Autodesk Fusion 360 part; units mm, degrees
(part 3 of 3)
ref_plane "Piano di lavoro7" through (0, 0, 107.5) normal (0, 0, 1) x (1, 0, 0) in component "14_Guscio_mobile_cannone_removibile"
sketch "Schizzo12 (5)" plane through (0, 0, 107.5) normal (0, 0, 1) x (1, 0, 0) in component "14_Guscio_mobile_cannone_removibile"
  line L0 (-15, -13) -> (15, -13)
  line L1 (15, -13) -> (15, 2)
  line L2 (15, 2) -> (-15, 2)
  line L3 (-15, 2) -> (-15, -13)
extrude "Tasca_coperchio_culatta_a_filo" cut sketch "Schizzo12 (5)" along normal blind 2 bodies 30 in component "14_Guscio_mobile_cannone_removibile"
ref_plane "Piano di lavoro8" through (0, -6, 0) normal (0, 1, 0) x (0, 0, 1) in component "14_Guscio_mobile_cannone_removibile"
sketch "Schizzo13 (5)" plane through (0, -6, 0) normal (0, 1, 0) x (1, 0, 0) in component "14_Guscio_mobile_cannone_removibile"
  circle A0 centre (0, -96.5) radius 5.5
extrude "Estrusione_Guida_interna_culatta_manuale" add sketch "Schizzo13 (5)" along normal blind 8 separate body makes body 33 in component "14_Guscio_mobile_cannone_removibile"
ref_plane "Piano di lavoro9" through (0, -6, 0) normal (0, 1, 0) x (0, 0, 1) in component "14_Guscio_mobile_cannone_removibile"
sketch "Schizzo14 (5)" plane through (0, -6, 0) normal (0, 1, 0) x (1, 0, 0) in component "14_Guscio_mobile_cannone_removibile"
  circle A0 centre (0, -96.5) radius 4
extrude "Foro_coassiale_guida_culatta_manuale" cut sketch "Schizzo14 (5)" along normal blind 8 bodies 33 in component "14_Guscio_mobile_cannone_removibile"
ref_plane "Piano di lavoro10" through (0, 0, 100.8) normal (0, 0, 1) x (1, 0, 0) in component "14_Guscio_mobile_cannone_removibile"
sketch "Schizzo15 (5)" plane through (0, 0, 100.8) normal (0, 0, 1) x (1, 0, 0) in component "14_Guscio_mobile_cannone_removibile"
  line L0 (-2, -6) -> (2, -6)
  line L1 (2, -6) -> (2, 2)
  line L2 (2, 2) -> (-2, 2)
  line L3 (-2, 2) -> (-2, -6)
extrude "Estrusione_Nervatura_tetto_guida_culatta" add sketch "Schizzo15 (5)" along normal blind 6.4 bodies 30 33 in component "14_Guscio_mobile_cannone_removibile"
ref_plane "Piano di lavoro11" through (0, 0, 103) normal (0, 0, 1) x (1, 0, 0) in component "14_Guscio_mobile_cannone_removibile"
sketch "Schizzo16 (4)" plane through (0, 0, 103) normal (0, 0, 1) x (1, 0, 0) in component "14_Guscio_mobile_cannone_removibile"
  circle A0 centre (-10.75, -4) radius 3
extrude "Estrusione_Boss_M2_5_coperchio_culatta_01" add sketch "Schizzo16 (4)" along normal blind 4.2 bodies 30 in component "14_Guscio_mobile_cannone_removibile"
sketch "Schizzo17 (3)" plane through (0, 0, 103) normal (0, 0, 1) x (1, 0, 0) in component "14_Guscio_mobile_cannone_removibile"
  circle A0 centre (-10.75, -4) radius 1.1
extrude "Preforo_M2_5_coperchio_culatta_01" cut sketch "Schizzo17 (3)" along normal blind 4.6 bodies 30 in component "14_Guscio_mobile_cannone_removibile"
sketch "Schizzo18 (3)" plane through (0, 0, 103) normal (0, 0, 1) x (1, 0, 0) in component "14_Guscio_mobile_cannone_removibile"
  circle A0 centre (10.75, -4) radius 3
extrude "Estrusione_Boss_M2_5_coperchio_culatta_02" add sketch "Schizzo18 (3)" along normal blind 4.2 bodies 30 in component "14_Guscio_mobile_cannone_removibile"
sketch "Schizzo19 (3)" plane through (0, 0, 103) normal (0, 0, 1) x (1, 0, 0) in component "14_Guscio_mobile_cannone_removibile"
  circle A0 centre (10.75, -4) radius 1.1
extrude "Preforo_M2_5_coperchio_culatta_02" cut sketch "Schizzo19 (3)" along normal blind 4.6 bodies 30 in component "14_Guscio_mobile_cannone_removibile"
sketch "Schizzo20 (3)" plane through (0, 0, 83.5) normal (0, 0, 1) x (1, 0, 0) in component "14_Guscio_mobile_cannone_removibile"
  line L0 (-28, 40.5) -> (-5.5, 40.5)
  line L1 (-5.5, 40.5) -> (-5.5, 43)
  line L2 (-5.5, 43) -> (-28, 43)
  line L3 (-28, 43) -> (-28, 40.5)
extrude "Estrusione_Parete_mobile_Anteriore_Ovest" add sketch "Schizzo20 (3)" along normal blind 26 bodies 30 in component "14_Guscio_mobile_cannone_removibile"
sketch "Schizzo21 (3)" plane through (0, 0, 83.5) normal (0, 0, 1) x (1, 0, 0) in component "14_Guscio_mobile_cannone_removibile"
  line L0 (5.5, 40.5) -> (28, 40.5)
  line L1 (28, 40.5) -> (28, 43)
  line L2 (28, 43) -> (5.5, 43)
  line L3 (5.5, 43) -> (5.5, 40.5)
extrude "Estrusione_Parete_mobile_Anteriore_Est" add sketch "Schizzo21 (3)" along normal blind 26 bodies 30 in component "14_Guscio_mobile_cannone_removibile"
ref_plane "Piano di lavoro12" through (0, 0, 102) normal (0, 0, 1) x (1, 0, 0) in component "14_Guscio_mobile_cannone_removibile"
sketch "Schizzo22 (3)" plane through (0, 0, 102) normal (0, 0, 1) x (1, 0, 0) in component "14_Guscio_mobile_cannone_removibile"
  line L0 (-5.5, 40.5) -> (5.5, 40.5)
  line L1 (5.5, 40.5) -> (5.5, 43)
  line L2 (5.5, 43) -> (-5.5, 43)
  line L3 (-5.5, 43) -> (-5.5, 40.5)
extrude "Estrusione_Ponte_superiore_cava_U_canna" add sketch "Schizzo22 (3)" along normal blind 7.5 bodies 30 in component "14_Guscio_mobile_cannone_removibile"
ref_plane "Piano di lavoro13" through (0, -13, 0) normal (0, 1, 0) x (0, 0, 1) in component "14_Guscio_mobile_cannone_removibile"
sketch "Schizzo23 (3)" plane through (0, -13, 0) normal (0, 1, 0) x (1, 0, 0) in component "14_Guscio_mobile_cannone_removibile"
  line L0 (-3, -83.5) -> (3, -83.5)
  line L1 (3, -83.5) -> (3, -87.5)
  line L2 (3, -87.5) -> (-3, -87.5)
  line L3 (-3, -87.5) -> (-3, -83.5)
extrude "Tacca_posteriore_cavo_cannone_aperta_inferiormente" cut sketch "Schizzo23 (3)" along normal blind 2.5 bodies 30 in component "14_Guscio_mobile_cannone_removibile"
ref_plane "Piano di lavoro14" through (0, 0, 85.5) normal (0, 0, 1) x (1, 0, 0) in component "14_Guscio_mobile_cannone_removibile"
sketch "Schizzo24 (3)" plane through (0, 0, 85.5) normal (0, 0, 1) x (1, 0, 0) in component "14_Guscio_mobile_cannone_removibile"
  circle A0 centre (-20, -5) radius 5
extrude "Estrusione_Colonna_M3_guscio_mobile_01" add sketch "Schizzo24 (3)" along normal blind 21.7 bodies 30 in component "14_Guscio_mobile_cannone_removibile"
sketch "Schizzo25 (3)" plane through (0, 0, 85.5) normal (0, 0, 1) x (1, 0, 0) in component "14_Guscio_mobile_cannone_removibile"
  circle A0 centre (-20, -5) radius 1.75
extrude "Foro_M3_guscio_mobile_01" cut sketch "Schizzo25 (3)" along normal blind 24 bodies 30 in component "14_Guscio_mobile_cannone_removibile"
sketch "Schizzo26 (3)" plane through (0, 0, 85.5) normal (0, 0, 1) x (1, 0, 0) in component "14_Guscio_mobile_cannone_removibile"
  circle A0 centre (20, -5) radius 5
extrude "Estrusione_Colonna_M3_guscio_mobile_02" add sketch "Schizzo26 (3)" along normal blind 21.7 bodies 30 in component "14_Guscio_mobile_cannone_removibile"
sketch "Schizzo27 (3)" plane through (0, 0, 85.5) normal (0, 0, 1) x (1, 0, 0) in component "14_Guscio_mobile_cannone_removibile"
  circle A0 centre (20, -5) radius 1.75
extrude "Foro_M3_guscio_mobile_02" cut sketch "Schizzo27 (3)" along normal blind 24 bodies 30 in component "14_Guscio_mobile_cannone_removibile"
sketch "Schizzo28 (3)" plane through (0, 0, 85.5) normal (0, 0, 1) x (1, 0, 0) in component "14_Guscio_mobile_cannone_removibile"
  circle A0 centre (-20, 35) radius 5
extrude "Estrusione_Colonna_M3_guscio_mobile_03" add sketch "Schizzo28 (3)" along normal blind 21.7 bodies 30 in component "14_Guscio_mobile_cannone_removibile"
sketch "Schizzo29 (3)" plane through (0, 0, 85.5) normal (0, 0, 1) x (1, 0, 0) in component "14_Guscio_mobile_cannone_removibile"
  circle A0 centre (-20, 35) radius 1.75
extrude "Foro_M3_guscio_mobile_03" cut sketch "Schizzo29 (3)" along normal blind 24 bodies 30 in component "14_Guscio_mobile_cannone_removibile"
sketch "Schizzo30 (3)" plane through (0, 0, 85.5) normal (0, 0, 1) x (1, 0, 0) in component "14_Guscio_mobile_cannone_removibile"
  circle A0 centre (20, 35) radius 5
extrude "Estrusione_Colonna_M3_guscio_mobile_04" add sketch "Schizzo30 (3)" along normal blind 21.7 bodies 30 in component "14_Guscio_mobile_cannone_removibile"
sketch "Schizzo31 (3)" plane through (0, 0, 85.5) normal (0, 0, 1) x (1, 0, 0) in component "14_Guscio_mobile_cannone_removibile"
  circle A0 centre (20, 35) radius 1.75
extrude "Foro_M3_guscio_mobile_04" cut sketch "Schizzo31 (3)" along normal blind 24 bodies 30 in component "14_Guscio_mobile_cannone_removibile"
ref_plane "Piano di lavoro1" through (0, 0, 107.5) normal (0, 0, 1) x (1, 0, 0) in component "15_Coperchio_culatta_L_removibile_M2_5"
sketch "Schizzo1 (23)" plane through (0, 0, 107.5) normal (0, 0, 1) x (1, 0, 0) in component "15_Coperchio_culatta_L_removibile_M2_5"
  line L0 (-14.7, -12.7) -> (14.7, -12.7)
  line L1 (14.7, -12.7) -> (14.7, 1.7)
  line L2 (14.7, 1.7) -> (-14.7, 1.7)
  line L3 (-14.7, 1.7) -> (-14.7, -12.7)
extrude "Estrusione_Piastra_superiore_coperchio_culatta_a_filo" add sketch "Schizzo1 (23)" along normal blind 1.8 separate body makes body 34 in component "15_Coperchio_culatta_L_removibile_M2_5"
ref_plane "Piano di lavoro2" through (0, -12.7, 0) normal (0, 1, 0) x (0, 0, 1) in component "15_Coperchio_culatta_L_removibile_M2_5"
sketch "Schizzo2 (22)" plane through (0, -12.7, 0) normal (0, 1, 0) x (1, 0, 0) in component "15_Coperchio_culatta_L_removibile_M2_5"
  line L0 (-6.7, -90.8) -> (6.7, -90.8)
  line L1 (6.7, -90.8) -> (6.7, -109.2)
  line L2 (6.7, -109.2) -> (-6.7, -109.2)
  line L3 (-6.7, -109.2) -> (-6.7, -90.8)
extrude "Estrusione_Piastra_posteriore_coperchio_culatta" add sketch "Schizzo2 (22)" along normal blind 1.9 bodies 34 in component "15_Coperchio_culatta_L_removibile_M2_5"
ref_plane "Piano di lavoro3" through (0, 0, 108.1) normal (0, 0, 1) x (1, 0, 0) in component "15_Coperchio_culatta_L_removibile_M2_5"
ref_plane "Piano di lavoro4" through (0, 0, 109.3) normal (0, 0, 1) x (1, 0, 0) in component "15_Coperchio_culatta_L_removibile_M2_5"
sketch "Schizzo3 (21)" plane through (0, 0, 107.5) normal (0, 0, 1) x (1, 0, 0) in component "15_Coperchio_culatta_L_removibile_M2_5"
  circle A0 centre (-10.75, -4) radius 1.35
extrude "Foro_M2_5_coperchio_culatta_01" cut sketch "Schizzo3 (21)" along normal blind 1.8 bodies 34 in component "15_Coperchio_culatta_L_removibile_M2_5"
sketch "Schizzo4 (20)" plane through (0, 0, 108.1) normal (0, 0, 1) x (1, 0, 0) in component "15_Coperchio_culatta_L_removibile_M2_5"
  circle A0 centre (-10.75, -4) radius 1.35
sketch "Schizzo5 (12)" plane through (0, 0, 109.3) normal (0, 0, 1) x (1, 0, 0) in component "15_Coperchio_culatta_L_removibile_M2_5"
  circle A0 centre (-10.75, -4) radius 2.5
loft "Svasatura_M2_5_coperchio_culatta_01" cut profiles "Schizzo4 (20)", "Schizzo5 (12)" section 1 section 2 bodies 34 in component "15_Coperchio_culatta_L_removibile_M2_5"
sketch "Schizzo6 (10)" plane through (0, 0, 107.5) normal (0, 0, 1) x (1, 0, 0) in component "15_Coperchio_culatta_L_removibile_M2_5"
  circle A0 centre (10.75, -4) radius 1.35
extrude "Foro_M2_5_coperchio_culatta_02" cut sketch "Schizzo6 (10)" along normal blind 1.8 bodies 34 in component "15_Coperchio_culatta_L_removibile_M2_5"
sketch "Schizzo7 (8)" plane through (0, 0, 108.1) normal (0, 0, 1) x (1, 0, 0) in component "15_Coperchio_culatta_L_removibile_M2_5"
  circle A0 centre (10.75, -4) radius 1.35
sketch "Schizzo8 (8)" plane through (0, 0, 109.3) normal (0, 0, 1) x (1, 0, 0) in component "15_Coperchio_culatta_L_removibile_M2_5"
  circle A0 centre (10.75, -4) radius 2.5
loft "Svasatura_M2_5_coperchio_culatta_02" cut profiles "Schizzo7 (8)", "Schizzo8 (8)" section 1 section 2 bodies 34 in component "15_Coperchio_culatta_L_removibile_M2_5"
sketch "Schizzo1 (24)" plane through (0, 0, 0) normal (0, 1, 0) x (1, 0, 0)
  line L0 (0, -20) -> (0, 20)
ref_plane "Piano di lavoro1" through (0, 0, 81.5) normal (0, 0, 1) x (1, 0, 0)
sketch "Schizzo2 (23)" plane through (0, 0, 81.5) normal (0, 0, 1) x (1, 0, 0)
  line L0 (-20, 0) -> (20, 0)
component "01_Tetto_elettronica_removibile" placed x (1, 0, 0) y (0, 1, 0) z (0, 0, 1) at (0, 0, 0)
component "02A_Rondella_assiale_torretta_sostituibile" placed x (1, 0, 0) y (0, 1, 0) z (0, 0, 1) at (0, 0, 0)
component "02_Stepper_28BYJ48_statore_fisso_riferimento" placed x (1, 0, 0) y (0, 1, 0) z (0, 0, 1) at (0, 0, 0)
component "02B_Rotore_albero_28BYJ48_riferimento" placed x (1, 0, 0) y (0, 1, 0) z (0, 0, 1) at (0, 0, 0)
component "03_Base_rotante_D100_sede_D_stepper" placed x (1, 0, 0) y (0, 1, 0) z (0, 0, 1) at (0, 0, 0)
component "03A_Fermaglio_anti_sollevamento_Est_M3" placed x (1, 0, 0) y (0, 1, 0) z (0, 0, 1) at (0, 0, 0)
component "03A_Fermaglio_anti_sollevamento_Ovest_M3" placed x (1, 0, 0) y (0, 1, 0) z (0, 0, 1) at (0, 0, 0)
component "03A_Fermaglio_anti_sollevamento_Nord_M3" placed x (1, 0, 0) y (0, 1, 0) z (0, 0, 1) at (0, 0, 0)
component "03A_Fermaglio_anti_sollevamento_Sud_M3" placed x (1, 0, 0) y (0, 1, 0) z (0, 0, 1) at (0, 0, 0)
component "04_Torretta_parte_fissa_azimut" placed x (1, 0, 0) y (0, 1, 0) z (0, 0, 1) at (0, 0, 0)
component "05_Servo_TowerPro_SG90_Sinistro_statore_riferimento" placed x (1, 0, 0) y (0, 1, 0) z (0, 0, 1) at (0, 0, 0)
component "06_Servo_TowerPro_SG90_Destro_statore_riferimento" placed x (1, 0, 0) y (0, 1, 0) z (0, 0, 1) at (0, 0, 0)
component "09_Torretta_parte_mobile_elevazione" placed x (1, 0, 0) y (0, 1, 0) z (0, 0, 1) at (0, 0, 0)
component "07_Albero_e_cornetto_croce_SG90_Sinistro_riferimento" placed x (1, 0, 0) y (0, 1, 0) z (0, 0, 1) at (0, 0, 0)
component "08_Albero_e_cornetto_croce_SG90_Destro_riferimento" placed x (1, 0, 0) y (0, 1, 0) z (0, 0, 1) at (0, 0, 0)
component "09A_Guancia_cornetto_Sinistra_regolabile" placed x (1, 0, 0) y (0, 1, 0) z (0, 0, 1) at (0, 0, 0)
component "09B_Guancia_cornetto_Destra_regolabile" placed x (1, 0, 0) y (0, 1, 0) z (0, 0, 1) at (0, 0, 0)
component "10_Modulo_cannone_reale_PCB_solenoide_canna" placed x (1, 0, 0) y (0, 1, 0) z (0, 0, 1) at (0, 0, 0)
component "11_Guscio_fisso_posteriore_torretta_removibile" placed x (1, 0, 0) y (0, 1, 0) z (0, 0, 1) at (0, 0, 0)
component "12_Carter_SG90_Sinistro_removibile" placed x (1, 0, 0) y (0, 1, 0) z (0, 0, 1) at (0, 0, 0)
component "13_Carter_SG90_Destro_removibile" placed x (1, 0, 0) y (0, 1, 0) z (0, 0, 1) at (0, 0, 0)
component "14_Guscio_mobile_cannone_removibile" placed x (1, 0, 0) y (0, 1, 0) z (0, 0, 1) at (0, 0, 0)
component "15_Coperchio_culatta_L_removibile_M2_5" placed x (1, 0, 0) y (0, 1, 0) z (0, 0, 1) at (0, 0, 0)
equation "cop_lunghezza = 176.0 mm" comment "Ingombro coperchio"
equation "cop_larghezza = 166.0 mm" comment "Ingombro coperchio"
equation "cop_parete_altezza = 30.0 mm" comment "Quota locale del tetto removibile"
equation "cop_tetto_spessore = 3.0 mm" comment "Coperchio elettronica"
equation "cop_boss_M3_diametro = 10.0 mm" comment "Accesso vite M3 dal tetto alle colonnine"
equation "cop_canale_fondo_raggio_interno = 19.0 mm" comment "Fondo liscio pista cavi tipo clock-spring"
equation "cop_canale_fondo_raggio_esterno = 40.0 mm" comment "Fondo liscio pista cavi tipo clock-spring"
equation "cop_canale_fondo_quota = 20.0 mm" comment "Quota locale fondo pista cavi"
equation "cop_canale_fondo_spessore = 3.0 mm" comment "Fondo strutturale pista cavi"
equation "cop_canale_parete_spessore = 1.5 mm" comment "Pareti lisce pista cavi"
equation "cop_canale_altezza_libera = 7.0 mm" comment "Altezza libera pista cavi"
equation "stepper_corpo_diametro = 28.0 mm" comment "Riferimento stepper"
equation "stepper_corpo_altezza = 20.0 mm" comment "Riferimento stepper"
equation "stepper_albero_diametro = 5.0 mm" comment "Riferimento stepper"
equation "stepper_albero_quota_tra_piatti = 3.0 mm" comment "Profilo doppia-D confermato"
equation "stepper_albero_lunghezza = 6.0 mm" comment "Riferimento stepper"
equation "stepper_interasse_fori = 35.0 mm" comment "Fissaggio stepper"
equation "stepper_foro_fissaggio = 4.2 mm" comment "Fissaggio stepper"
equation "stepper_svasatura_M4_diametro = 8.4 mm" comment "Testa svasata a filo"
equation "stepper_svasatura_M4_profondita = 2.1 mm" comment "Testa svasata a filo"
equation "torre_base_diametro = 100.0 mm" comment "Adattatore rotante"
equation "torre_base_spessore = 6.0 mm" comment "Adattatore rotante"
equation "torre_sede_D_diametro = 5.4 mm" comment "Mozzo D stepper"
equation "torre_sede_D_quota_tra_piatti = 3.4 mm" comment "Mozzo doppia-D stepper"
equation "torre_mozzo_accoppiamento_diametro = 12.0 mm" comment "Mozzo inferiore nel tetto"
equation "torre_mozzo_accoppiamento_altezza = 2.0 mm" comment "Impegno albero da 6 mm"
equation "torre_mozzo_gioco_tetto = 0.25 mm" comment "Gioco radiale per lato"
equation "torre_rondella_assiale_DI = 76.0 mm" comment "Appoggio assiale esterno ai cavi"
equation "torre_rondella_assiale_DE = 94.0 mm" comment "Appoggio assiale esterno ai cavi"
equation "torre_rondella_assiale_spessore = 0.8 mm" comment "Appoggio assiale esterno ai cavi"
equation "torre_rondella_sede_profondita = 0.3 mm" comment "Localizzazione rondella"
equation "torre_rondella_sede_gioco = 0.2 mm" comment "Gioco per lato sede rondella"
equation "torre_guida_fissa_RI = 34.5 mm" comment "Centraggio radiale"
equation "torre_guida_fissa_RE = 36.5 mm" comment "Centraggio radiale"
equation "torre_guida_fissa_altezza = 2.6 mm" comment "Centraggio radiale"
equation "torre_gola_gioco_radiale = 0.3 mm" comment "Gioco per lato"
equation "torre_gola_profondita = 2.5 mm" comment "Guida rotante"
equation "torre_fermaglio_gioco_verticale = 0.4 mm" comment "Anti-sollevamento"
equation "torre_fermaglio_sovrapposizione = 1.5 mm" comment "Anti-sollevamento"
equation "torre_fermaglio_foro_M3 = 3.2 mm" comment "Fermagli removibili"
equation "torre_fermaglio_spallamento_altezza = 1.5 mm" comment "Antirotazione fermagli"
equation "torre_fermaglio_spallamento_larghezza = 2.0 mm" comment "Antirotazione fermagli"
equation "torre_distanziale_telaio_altezza = 6.0 mm" comment "Evita collisione con fermagli"
equation "torre_distanziale_telaio_diametro = 10.0 mm" comment "Quattro appoggi M3"
equation "torre_fissa_larghezza = 80.0 mm" comment "Parte fissa torretta"
equation "torre_fissa_lunghezza = 70.0 mm" comment "Parte fissa torretta"
equation "torre_fissa_altezza = 50.0 mm" comment "Parte fissa torretta"
equation "torre_parete_spessore = 4.0 mm" comment "Parte fissa torretta"
equation "torre_perno_quota = 32.0 mm" comment "Asse elevazione"
equation "servo_corpo_lunghezza = 22.7 mm" comment "TowerPro SG90"
equation "servo_corpo_larghezza = 12.2 mm" comment "TowerPro SG90"
equation "servo_corpo_altezza = 27.0 mm" comment "TowerPro SG90"
equation "servo_ingombro_con_uscita = 30.3 mm" comment "TowerPro SG90"
equation "servo_alette_lunghezza_totale = 32.3 mm" comment "TowerPro SG90"
equation "servo_aletta_sporgenza = 5.0 mm" comment "Quota utente circa 5 mm"
equation "servo_aletta_spessore = 2.0 mm" comment "Quota utente 2 mm"
equation "servo_aletta_foro_M2_5 = 2.5 mm" comment "M2.5 provata sul pezzo"
equation "servo_aletta_asola_telaio_lunghezza = 5.0 mm" comment "Registrazione lungo Y"
equation "servo_aletta_asola_telaio_larghezza = 2.9 mm" comment "Passaggio M2.5 con gioco"
equation "servo_aletta_parete_minima = 1.2 mm" comment "Tra asola e finestra corpo"
equation "servo_asse_da_estremita = 17.0 mm" comment "TowerPro SG90"
equation "servo_albero_sporgenza = 3.3 mm" comment "TowerPro SG90"
equation "servo_albero_diametro_riferimento = 6.0 mm" comment "Solo inviluppo uscita SG90"
equation "servo_cornetto_span_riferimento = 33.0 mm" comment "Cornetto reale usato come dima"
equation "servo_cornetto_spessore_riferimento = 1.5 mm" comment "Quota visiva provvisoria"
equation "servo_adattatore_cornetto_diametro = 34.0 mm" comment "Disco pieno senza interassi inventati"
equation "servo_adattatore_cornetto_spessore = 4.0 mm" comment "Impegno viti appuntite"
equation "servo_adattatore_accesso_vite_centrale = 10.0 mm" comment "Accesso alla vite originale"
equation "servo_adattatore_asola_regolazione = 5.0 mm" comment "Registrazione assiale"
equation "servo_gioco_inserimento = 0.5 mm" comment "Slitta servo"
equation "servo_supporto_parete = 2.5 mm" comment "Slitta servo"
equation "servo_supporto_ripiano = 2.5 mm" comment "Slitta servo"
equation "servo_carter_foro_M2_5 = 2.7 mm" comment "Carter removibile"
equation "servo_carter_preforo_M2_5 = 2.2 mm" comment "Supporto carter"
equation "servo_cavo_larghezza = 4.0 mm" comment "Cavo piatto SG90"
equation "servo_cavo_spessore = 1.0 mm" comment "Cavo piatto SG90"
equation "servo_uscita_cavo_larghezza = 5.0 mm" comment "Slitta SG90"
equation "servo_uscita_cavo_profondita = 2.0 mm" comment "Slitta SG90"
equation "servo_connettore_larghezza = 7.0 mm" comment "Connettore SG90"
equation "servo_connettore_spessore = 3.0 mm" comment "Connettore SG90"
equation "passaggio_comune_larghezza = 9.0 mm" comment "Passaggio connettori SG90"
equation "passaggio_comune_lunghezza = 7.0 mm" comment "Passaggio connettori SG90"
equation "passaggio_arco_raggio = 28.0 mm" comment "Guida cavi azimut"
equation "passaggio_arco_larghezza = 9.0 mm" comment "Guida cavi azimut"
equation "ansa_azimut_lunghezza_libera = 210.0 mm" comment "Fascio ordinato nel canale"
equation "asola_fascetta_cavi_lunghezza = 5.0 mm" comment "Fermacavi torretta"
equation "asola_fascetta_cavi_larghezza = 2.0 mm" comment "Fermacavi torretta"
equation "asola_fascetta_cavi_interasse = 7.0 mm" comment "Fermacavi torretta"
equation "asola_fascetta_cannone_mobile_interasse = 12.0 mm" comment "Ancoraggio ansa elevazione"
equation "fermacavo_fisso_inferiore_larghezza = 18.0 mm" comment "Scarico trazione sotto uscita"
equation "fermacavo_fisso_inferiore_lunghezza = 12.0 mm" comment "Scarico trazione sotto uscita"
equation "fermacavo_fisso_inferiore_spessore = 2.0 mm" comment "Scarico trazione sotto uscita"
equation "fermacavo_fisso_asole_offset_x = 1.5 mm" comment "Sposta le asole fuori dal bordo anulare"
equation "fermacavo_fisso_ponte_larghezza = 20.0 mm" comment "Ponte strutturale verso il fondo anulare"
equation "fermacavo_fisso_ponte_lunghezza = 4.0 mm" comment "Ponte strutturale verso il fondo anulare"
equation "cannone_connettore_larghezza = 5.0 mm" comment "Connettore cannone"
equation "cannone_connettore_spessore = 3.0 mm" comment "Connettore cannone"
equation "cannone_passaggio_mobile_larghezza = 6.0 mm" comment "Passaggio sotto culla"
equation "cannone_passaggio_mobile_lunghezza = 4.0 mm" comment "Passaggio sotto culla"
equation "pcb_cannone_lunghezza = 50.0 mm" comment "PCB mobile cannone"
equation "pcb_cannone_larghezza = 50.0 mm" comment "PCB mobile cannone"
equation "pcb_cannone_spessore = 2.0 mm" comment "PCB mobile cannone"
equation "pcb_cannone_foro = 3.5 mm" comment "Fori PCB cannone"
equation "pcb_cannone_foro_bordo_x = 5.0 mm" comment "Fori PCB cannone"
equation "pcb_cannone_foro_bordo_y = 5.0 mm" comment "Fori PCB cannone"
equation "solenoide_diametro = 20.0 mm" comment "Zona solenoide"
equation "solenoide_lunghezza = 25.0 mm" comment "Zona solenoide"
equation "canna_diametro_esterno = 10.0 mm" comment "Canna tubolare"
equation "canna_diametro_interno = 8.0 mm" comment "Canna tubolare"
equation "canna_parete = 1.0 mm" comment "Canna tubolare"
equation "canna_sporgenza = 46.0 mm" comment "Canna tubolare"
equation "modulo_cannone_altezza = 23.0 mm" comment "Modulo mobile"
equation "culatta_proiettile_diametro_max_provvisorio = 7.0 mm" comment "Solo proiettile morbido e inerte"
equation "culatta_proiettile_lunghezza_max_provvisoria = 10.0 mm" comment "Ingombro di caricamento da verificare"
equation "culatta_guida_diametro_esterno = 11.0 mm" comment "Invito interno coassiale"
equation "culatta_guida_diametro_interno = 8.0 mm" comment "Invito interno coassiale"
equation "culatta_guida_lunghezza = 8.0 mm" comment "Invito interno coassiale"
equation "culatta_finestra_posteriore_larghezza = 14.0 mm" comment "Apertura a L removibile"
equation "culatta_asola_tetto_lunghezza = 12.0 mm" comment "Apertura a L removibile"
equation "culatta_coperchio_larghezza = 30.0 mm" comment "Coperchio a filo removibile"
equation "culatta_coperchio_lunghezza = 15.0 mm" comment "Coperchio a filo removibile"
equation "culatta_tasca_profondita = 2.0 mm" comment "Alloggiamento coperchio removibile"
equation "culatta_coperchio_spessore = 1.8 mm" comment "Coperchio a filo removibile"
equation "culatta_coperchio_gioco_verticale = 0.2 mm" comment "Coperchio leggermente ribassato"
equation "culatta_rinforzo_locale_spessore = 0.8 mm" comment "Rinforzo a U sotto la tasca"
equation "culatta_interasse_M2_5 = 21.5 mm" comment "Due viti accessibili dall'alto"
equation "culatta_foro_M2_5 = 2.7 mm" comment "Coperchio removibile"
equation "culatta_preforo_M2_5 = 2.2 mm" comment "Boss sotto il tetto"
equation "cannone_elevazione_min = -10.0 deg" comment "Limite proposto asse elevazione"
equation "cannone_elevazione_max = 35.0 deg" comment "Limite proposto asse elevazione"
equation "passaggio_arco_angolo_iniziale = 0.0 deg" comment "Inizio guida cavi di azimut"
equation "passaggio_arco_corsa = 360.0 deg" comment "Corsa totale guida cavi di azimut"
equation "torretta_azimut_min = -180.0 deg" comment "Limite software e giunto Fusion"
equation "torretta_azimut_max = 180.0 deg" comment "Limite software e giunto Fusion"
equation "d135 = cop_parete_altezza"
equation "d137 = cop_tetto_spessore"
equation "d155 = cop_parete_altezza"
equation "d161 = cop_tetto_spessore"
equation "d163 = cop_tetto_spessore"
equation "d165 = cop_tetto_spessore"
equation "d167 = cop_tetto_spessore"
equation "d171 = cop_tetto_spessore"
equation "d175 = cop_tetto_spessore"
equation "d179 = cop_tetto_spessore"
equation "d191 = cop_canale_fondo_spessore"
equation "d193 = cop_canale_fondo_spessore"
equation "d205 = cop_tetto_spessore"
equation "d239 = stepper_corpo_altezza"
equation "d247 = stepper_albero_lunghezza"
equation "d249 = stepper_albero_lunghezza"
equation "d251 = stepper_albero_lunghezza"
equation "d255 = torre_base_spessore"
equation "d275 = torre_base_spessore"
equation "d279 = torre_base_spessore"
equation "d283 = torre_base_spessore"
equation "d287 = torre_base_spessore"
equation "d291 = torre_base_spessore"
equation "d483 = servo_corpo_altezza"
equation "d499 = servo_corpo_altezza"
equation "d621 = pcb_cannone_spessore"
equation "d623 = pcb_cannone_spessore"
equation "d625 = pcb_cannone_spessore"
equation "d627 = pcb_cannone_spessore"
equation "d629 = pcb_cannone_spessore"
equation "d637 = solenoide_lunghezza"
equation "d641 = solenoide_lunghezza"
equation "d645 = canna_sporgenza"
equation "d649 = canna_sporgenza"
equation "guscio_torretta_parete = 2.5 mm" comment "Gusci removibili torretta"
equation "guscio_torretta_gioco = 0.5 mm" comment "Gioco attorno a telaio, servo e modulo mobile"
equation "guscio_cannone_foro_canna = 11.0 mm" comment "Passaggio canna nel guscio mobile"
named bodies: "Tetto_fisso_canale_cavi_guida_radiale_supporto_stepper_boss_M3", "Labbro_fisso_centraggio_radiale_torretta", "Rondella_assiale_DI76_DE94_spessore_0_8", "Corpo_stepper", "Albero_stepper", "Base_rotante_D100_sede_D_gola_guida_passaggio_cavi", "Piede_fermaglio_Est", "Piede_fermaglio_Ovest", "Piede_fermaglio_Nord", "Piede_fermaglio_Sud", "Base_parte_fissa", "Corpo_SG90_Sinistro", "Corpo_SG90_Destro", "Piastra_culla_mobile", "Albero_uscita_SG90_Sinistro", "Cornetto_croce_orizzontale_Sinistro", "Albero_uscita_SG90_Destro", "Cornetto_croce_orizzontale_Destro", "Disco_pieno_cornetto_Sinistra", "Mensola_sotto_culla_Sinistra", "Disco_pieno_cornetto_Destra", "Mensola_sotto_culla_Destra", "PCB_modulo_cannone_50x50", "Appoggio_solenoide_su_PCB", "Corpo_solenoide_riferimento", "Canna_tubolare_esterna", "Parete_posteriore_guscio_torretta", "Parete_esterna_carter_Sinistro", "Parete_esterna_carter_Destro", "Parete_mobile_Ovest", "Disco_pieno_cornetto_Sinistra (1)", "Disco_pieno_cornetto_Destra (1)", "Guida_interna_culatta_manuale", "Piastra_superiore_coperchio_culatta_a_filo"
